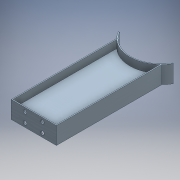
# Autodesk Inventor part: Fix Saddle Pervecto
Saved by Autodesk Inventor 2016 (Build 200138000, 138)
## iProperties
Created: 2018-11-07
Part Number: Fix Saddle Pervecto
Material: Steel ASTM A36
Document SubType Name: Modeling
Designer: asus
Density: 7.85 g/cm^3
Appearance: Steel Blue
Mass: 18212.1 g
Surface Area: 6484.58 cm^2
Volume: 2320.01 cm^3
Author: asus
Autodesk Inventor part; units mm, degrees
ref_plane "YZ Plane" through (0, 0, 0) normal (1, 0, 0) x (0, 1, 0)
ref_plane "XZ Plane" through (0, 0, 0) normal (0, 1, 0) x (-1, 0, 0)
ref_plane "XY Plane" through (0, 0, 0) normal (0, 0, 1) x (1, 0, 0)
sketch "Sketch1" plane through (0, 0, 0) normal (0, 0, 1) x (1, 0, 0)
  line L0 (-130, 607) -> (-130, 0)
  line L1 (-130, 0) -> (130, 0)
  line L2 (130, 0) -> (130, 607)
  line L3 (125, 5) -> (125, 602.1317)
  line L4 (-125, 5) -> (-125, 602.1317)
  line L5 (-125, 5) -> (125, 5)
  arc A0 (-153.9793, 646.614) -> (153.9793, 646.614) centre (0, 735.514) ccw
  arc A1 (130, 607) -> (158.3094, 644.114) centre (0, 735.514) ccw
  arc A2 (-158.3094, 644.114) -> (-130, 607) centre (0, 735.514) ccw
  arc A3 (-125, 602.1317) -> (125, 602.1317) centre (0, 735.514) ccw
  line L6 (-158.3094, 644.114) -> (-153.9793, 646.614)
  line L7 (153.9793, 646.614) -> (158.3094, 644.114)
  point P0 (0, 0)
  point P1 (0, 0)
  point P2 (0, 5)
  dimension "d0" = 260
  dimension "d2" = 607
  dimension "d3" = 607
  dimension "d6" = 5
  dimension "d7" = 5
  dimension "d8" = 5
  dimension "d57" = 355.6
  dimension "d61" = 5
  dimension "d64" = 182.8
  dimension "d79" = 130
  dimension "d80" = 120
  dimension "d81" = 158.3094
  dimension "d82" = 153.9793
  dimension "d83" = 153.9793
  constraints: 16 end point, 8 point on circle, 4 centre point, 4 coincident, 3 vertical, 2 midpoint, 2 perpendicular, 1 parallel, 1 vertical alignment
  measures "d0" distance of L0.end L1.end
  measures "d2" distance of L0.start L0.end
  measures "d3" distance of L1.end L2.end
  measures "d6" distance between parallel lines of L0 L4
  measures "d7" distance between parallel lines of L2 L3
  measures "d8" distance between parallel lines of L1 L5
  measures "d57" diameter of A0
  measures "d61" radial gap between concentric circles of A3 A0
  measures "d64" radius of A1
  measures "d79" distance from line of L0 A1.centre
  measures "d80" angle of L7 L6
  measures "d81" horizontal distance of L6.start A0.centre
  measures "d82" horizontal distance of L6.end A0.centre
  measures "d83" horizontal distance of L7.start A0.centre
extrude "Extrusion1" add sketch "Sketch1" along normal mid plane 100
sketch "Sketch5" plane through (0, 0, 0) normal (0, 0, 1) x (1, 0, 0)
  line L0 (-125, 602.1317) -> (-125, 5) projected
  line L1 (-125, 602.1317) -> (-125, 5)
  line L2 (-125, 5) -> (125, 5)
  line L3 (-125, 5) -> (125, 5) projected
  line L4 (125, 5) -> (125, 602.1317) projected
  line L5 (125, 5) -> (125, 602.1317)
  arc A0 (-125, 602.1317) -> (125, 602.1317) centre (0, 735.514) ccw
  point P0 (0, 0)
  point P1 (0, 5)
  dimension "d67" = 365.6
  constraints: 6 end point, 2 collinear, 2 perpendicular, 2 point on circle, 1 centre point, 1 midpoint, 1 vertical alignment
  measures "d67" diameter of A0
extrude "Extrusion2" add sketch "Sketch5" along normal mid plane 10
sketch "Sketch6" plane through (-130, 0, 50) normal (0, -1, 0) x (1, 0, 0)
  line L0 (5, -100) -> (255, -100) projected
  line L1 (130, -100) -> (130, 0)
  line L2 (0, 0) -> (260, 0) projected
  circle A0 centre (180, -77.5) radius 10
  circle A1 centre (180, -22.5) radius 10
  circle A2 centre (80, -77.5) radius 10
  circle A3 centre (80, -22.5) radius 10
  point P0 (130, -50)
  dimension "d72" = 20
  dimension "d73" = 100
  dimension "d74" = 20
  dimension "d75" = 55
  dimension "d76" = 100
  dimension "d84" = 22.5
  constraints: 4 centre point, 2 end point, 2 midpoint, 2 symmetric about line, 2 other
  measures "d72" diameter of A0
  measures "d73" diameter of A0.centre L1
  measures "d74" diameter of A1
  measures "d75" distance of A1.centre A0.centre
  measures "d76" diameter of A1.centre L1
  measures "d84" distance from line of L0 A0.centre
extrude "Extrusion5" cut sketch "Sketch6" against normal blind 10
body "Solid1"
